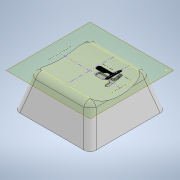
# Autodesk Inventor part: KeycapS
Saved by Autodesk Inventor 2022 (Build 260153000, 153)
## iProperties
Created: 2022-03-01
Part Number: KeycapS
Material: Generic
Document SubType Name: Modeling
Designer: Nathan Griffith
Density: 1 g/cm^3
Appearance: Default
Author: Nathan Griffith
Autodesk Inventor part; units mm, degrees
ref_plane "YZ Plane" through (0, 0, 0) normal (1, 0, 0) x (0, 1, 0)
ref_plane "XZ Plane" through (0, 0, 0) normal (0, 1, 0) x (-1, 0, 0)
ref_plane "XY Plane" through (0, 0, 0) normal (0, 0, 1) x (1, 0, 0)
sketch "Sketch1" plane through (0, 0, 0) normal (0, 1, 0) x (-1, 0, 0)
  line L0 (0, 0) -> (18, 0)
  line L1 (18, 0) -> (18, 18)
  line L2 (18, 18) -> (0, 18)
  line L3 (0, 18) -> (0, 0)
  dimension "d0" = 18
  dimension "d1" = 18
  constraints: 8 end point, 2 parallel, 1 horizontal, 1 perpendicular
  measures "d0" distance of L2.end L1.end
  measures "d1" distance of L1.end L0.end
extrude "Extrusion1" add sketch "Sketch1" along normal blind 8 draft -15
fillet "Fillet1" radius 1.5 8 edges at (-1.0718, 4, 16.9282) (-9, 8, 15.8564) (-2.1436, 8, 9) (-9, 8, 2.1436) (-1.0718, 4, 1.0718) (-16.9282, 4, 1.0718) (-16.9282, 4, 16.9282) (-15.8564, 8, 9)
ref_plane "Work Plane1" through (-9, 33.5885, 16.5511) normal (1, 0, 0) x (0, 0, -1)
sketch "Sketch2" plane through (-9, 33.5885, 16.5511) normal (1, 0, 0) x (0, 0, -1)
  line L0 (13.2565, -25.5885) -> (1.8457, -25.5885) projected
  arc A0 (14.7054, -26.7002) -> (13.2565, -25.5885) centre (13.2565, -27.0885) ccw projected
  arc A1 (1.8457, -25.5885) -> (13.2565, -25.5885) centre (7.5511, -15.0316) ccw
  point P0 (16.5511, -33.5885)
  point P1 (13.2565, -25.5885)
  dimension "d5" = 12
  constraints: 3 point on circle, 1 centre point
  measures "d5" radius of A1
extrude "Extrusion2" cut sketch "Sketch2" along normal through all both and the other way through all
sketch "Sketch3" plane through (0, 0, 0) normal (0, -1, 0) x (1, 0, 0)
  line L0 (-16.5511, 18) -> (-1.4489, 18) construction
  line L1 (-9, 18) -> (-9, 0) construction
  line L2 (-1.4489, 0) -> (-16.5511, 0) construction
  line L3 (-18, 1.4489) -> (-18, 16.5511) construction
  line L4 (-18, 9) -> (0, 9) construction
  line L5 (-1, 1) -> (-17, 1)
  line L6 (-17, 1) -> (-17, 17)
  line L7 (-17, 17) -> (-1, 17)
  line L8 (-1, 17) -> (-1, 1)
  line L9 (-1, 1) -> (-17, 17) construction
  line L10 (-17, 1) -> (-1, 17) construction
  point P0 (0, 0)
  point P1 (-9, 9)
  point P2 (-9, 9)
  dimension "d8" = 16
  dimension "d9" = 16
  constraints: 16 end point, 8 midpoint, 2 horizontal, 2 parallel, 1 perpendicular
  measures "d8" distance of L6.end L7.end
  measures "d9" distance of L7.end L5.start
extrude "Extrusion3" cut sketch "Sketch3" against normal blind 4.5 draft -15
sketch "Sketch4" plane through (0, 4.5, 0) normal (0, -1, 0) x (1, 0, 0)
  line L0 (-15.7942, 15.7942) -> (-15.7942, 2.2058) construction
  line L1 (-15.7942, 9) -> (-2.2058, 9) construction
  line L2 (-2.2058, 2.2058) -> (-2.2058, 15.7942) construction
  line L3 (-2.2058, 15.7942) -> (-15.7942, 15.7942) construction
  line L4 (-9, 15.7942) -> (-9, 2.2058) construction
  line L5 (-15.7942, 2.2058) -> (-2.2058, 2.2058) construction
  circle A0 centre (-9, 9) radius 2.775
  point P0 (0, 0)
  dimension "d12" = 5.55
  constraints: 5 midpoint, 4 end point, 1 centre point
  measures "d12" diameter of A0
extrude "Extrusion4" add sketch "Sketch4" along normal blind 4
sketch "Sketch5" plane through (-9, 0.5, 9) normal (0, -1, 0) x (1, 0, 0)
  line L0 (0.6, 2.075) -> (-0.6, 2.075)
  line L1 (-0.6, -2.075) -> (0.6, -2.075)
  line L2 (-0.6, 2.075) -> (0.6, -2.075) construction
  line L3 (-2.075, 0.6) -> (-2.075, -0.6)
  line L4 (2.075, -0.6) -> (2.075, 0.6)
  line L5 (2.075, 0.6) -> (-2.075, -0.6) construction
  line L6 (-2.075, 0.6) -> (2.075, -0.6) construction
  line L7 (-6.7942, 6.7942) -> (-6.7942, -6.7942) construction
  line L8 (-6.7942, 0) -> (6.7942, 0) construction
  line L9 (6.7942, -6.7942) -> (6.7942, 6.7942) construction
  line L10 (-6.7942, -6.7942) -> (6.7942, -6.7942) construction
  line L11 (0, -6.7942) -> (0, 6.7942) construction
  arc A0 (0.9, -0.6) -> (0.6, -0.9) centre (0.9, -0.9) ccw
  arc A1 (-0.6, -0.9) -> (-0.9, -0.6) centre (-0.9, -0.9) ccw
  arc A2 (0.6, 0.9) -> (0.9, 0.6) centre (0.9, 0.9) ccw
  arc A3 (-0.9, 0.6) -> (-0.6, 0.9) centre (-0.9, 0.9) ccw
  line L12 (-0.6, 2.075) -> (-0.6, 0.9)
  line L13 (-0.6, -0.9) -> (-0.6, -2.075)
  line L14 (-2.075, -0.6) -> (-0.9, -0.6)
  line L15 (-0.9, 0.6) -> (-2.075, 0.6)
  line L16 (0.6, 2.075) -> (0.1735, 0.6) construction
  line L17 (0, 0) -> (-0.6, -2.075) construction
  line L18 (2.075, 0.6) -> (0.9, 0.6)
  line L19 (0.9, -0.6) -> (2.075, -0.6)
  line L20 (0.6, -2.075) -> (0.6, -0.9)
  line L21 (0.6, 0.9) -> (0.6, 2.075)
  point P0 (9, -9)
  dimension "d15" = 1.2
  dimension "d16" = 4.15
  dimension "d17" = 4.15
  dimension "d18" = 1.2
  dimension "d19" = 0.3
  constraints: 38 end point, 10 parallel, 9 midpoint, 9 symmetric about line, 8 point on circle, 4 centre point, 4 perpendicular, 4 tangent, 3 horizontal, 1 vertical, 3 other
  measures "d15" distance of L1.end L1.start
  measures "d16" distance of L1.start L0.end
  measures "d17" distance of L4.start L3.end
  measures "d18" distance of L3.end L3.start
  measures "d19" radius of A0
extrude "Extrusion5" cut sketch "Sketch5" against normal blind 4
ref_plane "Work Plane2" through (-13.5, 8, 3.2946) normal (0, -1, 0) x (1, 0, 0)
sketch "Sketch6" plane through (-13.5, 8, 3.2946) normal (0, -1, 0) x (1, 0, 0)
  ellipse E0 centre (8.5277, 5.7054) end of major axis (8.5277, 17.7054) minor radius 3.2154 (11.6543, 2.9051) -> (11.6543, 8.5058) ccw construction
  line L0 (11.6543, 2.9051) -> (11.6543, 8.5058) construction
  ellipse E1 centre (0.4723, 5.7054) end of major axis (0.4723, -6.2946) minor radius 3.2154 (-2.6543, 8.5058) -> (-2.6543, 2.9051) ccw construction
  line L1 (-2.6543, 2.9051) -> (-2.6543, 8.5058) construction
  line L2 (11.6543, 5.7054) -> (4.4996, 5.8101) construction
  line L3 (-1.2054, 0) -> (10.2054, 0) construction
  line L4 (4.5, 0) -> (4.4996, 5.8101) construction
  line L5 (10.2054, 11.4108) -> (-1.2054, 11.4108) construction
  line L6 (4.4996, 5.8101) -> (4.5, 11.4108) construction
  line L7 (4.4996, 5.8101) -> (-2.6543, 5.7054) construction
  line L8 (4.4998, 2.9051) -> (11.6543, 2.9051) construction
  line L9 (8.077, 5.7578) -> (8.077, 0) construction
  spline S0 degree 2 poles (8.1996, 1.9165) (8.3005, 1.9165) (8.5025, 2.0745) (8.5024, 2.1832) knots 0 0 0 1 2 2 2
  line L10 (8.5024, 2.1832) -> (8.5178, 5.3392)
  spline S1 degree 2 poles (8.5178, 5.3392) (8.5178, 5.4091) (8.4763, 5.5515) (8.3961, 5.6706) (8.277, 5.7456) (8.1993, 5.7456) knots 0 0 0 1 2 3 4 4 4
  spline S2 degree 2 poles (8.1993, 5.7456) (8.1294, 5.7456) (8.0051, 5.6705) (7.9171, 5.5514) (7.8628, 5.409) (7.8628, 5.3391) knots 0 0 0 1 2 3 4 4 4
  line L11 (7.8628, 5.3391) -> (7.8628, 4.4641)
  spline S3 degree 2 poles (7.8628, 4.4641) (7.8628, 4.4278) (7.7981, 4.3268) (7.6971, 4.2388) (7.5962, 4.1741) (7.5625, 4.1741) knots 0 0 0 1 2 3 4 4 4
  line L12 (7.5625, 4.1741) -> (7.1586, 4.174)
  line L13 (7.1586, 4.174) -> (7.024, 4.2439)
  line L14 (7.024, 4.2439) -> (6.6227, 4.6219)
  spline S4 degree 2 poles (6.6227, 4.6219) (6.5735, 4.6633) (6.4078, 4.7125) (6.3508, 4.7125) knots 0 0 0 1 2 2 2
  line L15 (6.3508, 4.7125) -> (5.0071, 4.7124)
  spline S5 degree 2 poles (5.0071, 4.7124) (4.8829, 4.7124) (4.6939, 4.6062) (4.5774, 4.4328) (4.5178, 4.2153) (4.5179, 4.1091) knots 0 0 0 1 2 3 4 4 4
  spline S6 degree 2 poles (4.5179, 4.1091) (4.5179, 3.9435) (4.6059, 3.7001) (4.7431, 3.594) knots 0 0 0 1 2 2 2
  spline S7 degree 2 poles (4.7431, 3.594) (4.7664, 3.5758) (4.8674, 3.5189) (4.8778, 3.5189) knots 0 0 0 1 2 2 2
  line L16 (4.8778, 3.5189) -> (7.4719, 3.519)
  spline S8 degree 2 poles (7.4719, 3.519) (7.5134, 3.5191) (7.6506, 3.4595) (7.7749, 3.3586) (7.8629, 3.2472) (7.8629, 3.1929) knots 0 0 0 1 2 3 4 4 4
  line L17 (7.8629, 3.1929) -> (7.863, 2.3178)
  spline S9 degree 2 poles (7.863, 2.3178) (7.863, 2.2479) (7.9173, 2.1055) (8.0054, 1.9942) (8.1296, 1.9165) (8.1996, 1.9165) knots 0 0 0 1 2 3 4 4 4
  point P0 (13.5, -3.2946)
  constraints: 16 end point, 6 midpoint, 3 vertical, 1 horizontal, 1 point on line, 3 other
extrude "Extrusion6" cut sketch "Sketch6" along normal blind 1.6
body "Solid1"
